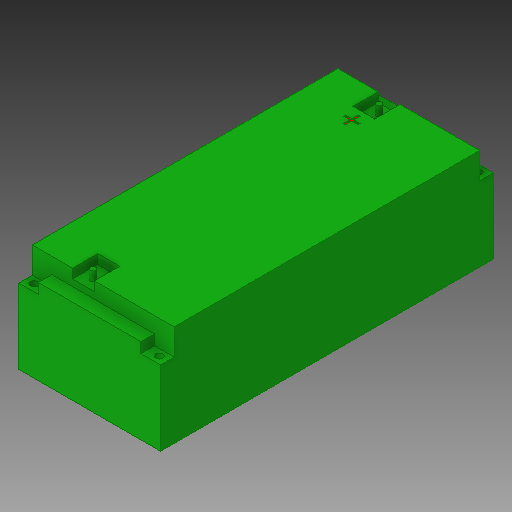
# Autodesk Inventor part: 47Ah-FoMoCo
Saved by Autodesk Inventor 2017 (Build 210142000, 142)
## iProperties
Created: 2022-08-13
Part Number: 47Ah-FoMoCo
Material: Generic
Document SubType Name: Modeling
Designer: JTS
Density: 1 g/cm^3
Appearance: Default
Author: JTS
Autodesk Inventor part; units mm, degrees
ref_plane "YZ Plane" through (0, 0, 0) normal (1, 0, 0) x (0, 1, 0)
ref_plane "XZ Plane" through (0, 0, 0) normal (0, 1, 0) x (-1, 0, 0)
sketch "Sketch1" plane through (0, 0, 0) normal (0, 1, 0) x (-1, 0, 0)
  line L0 (-75.875, 178) -> (75.875, 178)
  line L1 (75.875, 178) -> (75.875, -178)
  line L2 (75.875, -178) -> (-75.875, -178)
  line L3 (-75.875, -178) -> (-75.875, 178)
  line L4 (-75.875, 178) -> (75.875, -178) construction
  line L5 (75.875, 178) -> (-75.875, -178) construction
  circle A0 centre (67, 170.5) radius 4
  circle A1 centre (-67, 170.5) radius 4
  circle A2 centre (-67, -170.5) radius 4
  circle A3 centre (67, -170.5) radius 4
  line L6 (67, 170.5) -> (-67, 170.5) construction
  line L7 (75.875, 178) -> (67, 170.5) construction
  line L8 (-67, 170.5) -> (-75.875, 178) construction
  line L9 (67, -170.5) -> (67, 170.5) construction
  line L10 (67, -170.5) -> (-67, -170.5) construction
  line L11 (-67, -170.5) -> (-75.875, -178) construction
  line L12 (67, -170.5) -> (75.875, -178) construction
  point P0 (0, 0)
  dimension "d0" = 151.75
  dimension "d1" = 356
  dimension "d11" = 8
  dimension "d12" = 134
  dimension "d13" = 7.5
  constraints: 26 end point, 4 centre point, 4 horizontal, 3 equal length, 3 equal radius, 3 vertical, 2 midpoint
  measures "d0" distance of L1.end L2.end
  measures "d1" distance of L0.end L1.end
  measures "d11" diameter of A0
  measures "d12" distance of L6.start L6.end
  measures "d13" distance between parallel lines of L0 L6
extrude "Extrusion1" add sketch "Sketch1" along normal blind 108
sketch "Sketch2" plane through (0, 108, 0) normal (0, 1, 0) x (1, 0, 0)
  line L0 (-75.875, -178) -> (75.875, -178) projected
  line L1 (75.875, 178) -> (-75.875, 178) projected
  line L2 (-32.875, 178) -> (-32.875, 136.5)
  line L3 (-32.875, 136.5) -> (-9.375, 136.5)
  line L4 (-9.375, 136.5) -> (-9.375, 178)
  line L5 (-32.875, -178) -> (-32.875, -136.5)
  line L6 (-32.875, -136.5) -> (-9.375, -136.5)
  line L7 (-9.375, -136.5) -> (-9.375, -178)
  circle A0 centre (-21.125, -153) radius 3
  circle A1 centre (-21.125, 153) radius 3
  line L8 (-32.875, 178) -> (-21.125, 153) construction
  line L9 (-21.125, 153) -> (-9.375, 178) construction
  line L10 (-32.875, -178) -> (-21.125, -153) construction
  line L11 (-21.125, -153) -> (-9.375, -178) construction
  point P0 (0, 0)
  dimension "d4" = 43
  dimension "d5" = 23.5
  dimension "d6" = 41.5
  dimension "d19" = 6
  dimension "d20" = 25
  constraints: 20 end point, 5 point on line, 4 equal length, 4 vertical, 2 centre point, 2 horizontal, 1 collinear, 1 equal radius
  measures "d4" distance from line of L0.start L5
  measures "d5" distance of L5.end L6.end
  measures "d6" distance between parallel lines of L6 L0
  measures "d19" diameter of A0
  measures "d20" distance from line of L10.end L0
extrude "Extrusion2" cut sketch "Sketch2" against normal blind 10
sketch "Sketch3" plane through (0, 108, 0) normal (0, 1, 0) x (1, 0, 0)
  line L0 (-32.875, -178) -> (-32.875, -136.5) projected
  line L1 (-75.875, -178) -> (-32.875, -178) projected
  line L2 (-31.0347, 131.2602) -> (-10.3663, 131.2602) construction
  line L3 (-10.3663, 131.2602) -> (-10.3663, 113.395) construction
  line L4 (-10.3663, 113.395) -> (-31.0347, 113.395) construction
  line L5 (-31.0347, 113.395) -> (-31.0347, 131.2602) construction
  line L6 (-13.1255, 122.3299) -> (-19.9002, 122.3299)
  line L7 (-19.9002, 122.3299) -> (-19.9002, 115.5552)
  line L8 (-19.9002, 115.5552) -> (-22.1369, 115.5552)
  line L9 (-22.1369, 115.5552) -> (-22.1369, 122.3299)
  line L10 (-22.1369, 122.3299) -> (-28.9116, 122.3299)
  line L11 (-28.9116, 122.3299) -> (-28.9116, 124.4855)
  line L12 (-28.9116, 124.4855) -> (-22.1369, 124.4855)
  line L13 (-22.1369, 124.4855) -> (-22.1369, 131.2602)
  line L14 (-22.1369, 131.2602) -> (-19.9002, 131.2602)
  line L15 (-19.9002, 131.2602) -> (-19.9002, 124.4855)
  line L16 (-19.9002, 124.4855) -> (-13.1255, 124.4855)
  line L17 (-13.1255, 124.4855) -> (-13.1255, 122.3299)
  point P0 (0, 0)
  point P1 (-32.875, 178)
  point P2 (-75.875, 178)
  point P3 (-32.875, 136.5)
  constraints: 1 horizontal, 2 other
extrude "Extrusion3" cut sketch "Sketch3" against normal blind 1
ref_plane "Work Plane1" through (0, 80, 0) normal (0, -1, 0) x (1, 0, 0)
sketch "Sketch4" plane through (0, 108, 0) normal (0, 1, 0) x (1, 0, 0)
  line L0 (-75.875, -178) -> (-32.875, -178) projected
  line L1 (-75.875, 178) -> (-75.875, -178) projected
  line L2 (-9.375, -178) -> (75.875, -178) projected
  line L3 (75.875, -178) -> (75.875, 178) projected
  line L4 (75.875, 178) -> (-9.375, 178) projected
  line L5 (-32.875, 178) -> (-75.875, 178) projected
  line L6 (-75.875, 163.5) -> (-54.875, 163.5)
  line L7 (-54.875, 163.5) -> (-54.875, 178)
  line L8 (54.875, 178) -> (54.875, 163.5)
  line L9 (54.875, 163.5) -> (75.875, 163.5)
  line L10 (54.875, -178) -> (54.875, -163.5)
  line L11 (54.875, -163.5) -> (75.875, -163.5)
  line L12 (-54.875, -178) -> (-54.875, -163.5)
  line L13 (-54.875, -163.5) -> (-75.875, -163.5)
  point P0 (0, 0)
  dimension "d14" = 327
  dimension "d15" = 21
  constraints: 16 end point, 9 point on line, 6 collinear, 3 horizontal, 2 vertical
  measures "d14" distance between parallel lines of L6 L13
  measures "d15" distance between parallel lines of L1 L12
extrude "Extrusion4" cut sketch "Sketch4" against normal up to surface (28 mm away)
sketch "Sketch6" plane through (75.875, 0, 178) normal (1, 0, 0) x (0, 0, -1)
  line L0 (0, 80) -> (0, 108) projected
  line L1 (0, 108) -> (14.5, 108) projected
  line L2 (341.5, 108) -> (356, 108) projected
  line L3 (356, 108) -> (356, 80) projected
  line L4 (356, 0) -> (0, 0) construction
  line L5 (341.5, 108) -> (341.5, 80) projected
  line L6 (14.5, 108) -> (14.5, 80) projected
  line L7 (0, 91) -> (14.5, 91)
  line L8 (341.5, 91) -> (356, 91)
  point P0 (178, 0)
  dimension "d24" = 91
  constraints: 4 end point, 4 point on line, 1 collinear, 1 horizontal
  measures "d24" distance between parallel lines of L4 L7
extrude "Extrusion6" cut sketch "Sketch6" against normal up to surface (151.75 mm away)
body "Solid1"
